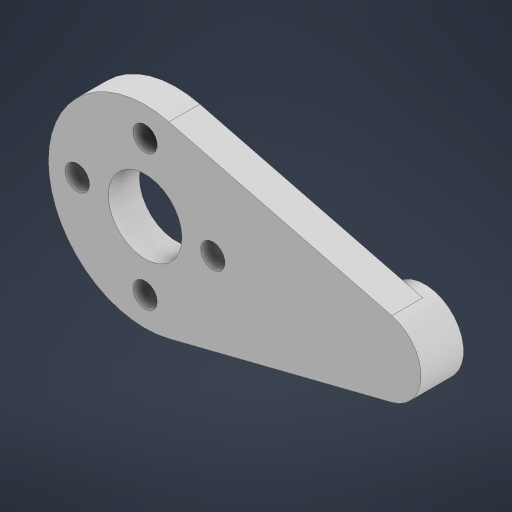
# Autodesk Inventor part: Magnet-arm
Saved by Autodesk Inventor 2024.2 (Build 282272000, 272)
## iProperties
Created: 2024-02-26
Part Number: Magnet-arm
Material: Generisch
Document SubType Name: Modeling
Designer: jacob
Density: 1 g/cm^3
Appearance: Vorgabe
Author: jacob
Autodesk Inventor part; units mm, degrees
ref_plane "YZ Plane" through (0, 0, 0) normal (1, 0, 0) x (0, 1, 0)
ref_plane "XZ Plane" through (0, 0, 0) normal (0, 1, 0) x (-1, 0, 0)
ref_plane "XY Plane" through (0, 0, 0) normal (0, 0, 1) x (1, 0, 0)
sketch "Skizze1" plane through (0, 0, 0) normal (0, 0, 1) x (1, 0, 0)
  arc A0 (2.449, 9.6955) -> (2.449, -9.6955) centre (0, 0) ccw
  arc A1 (25.4796, -3.8782) -> (25.4796, 3.8782) centre (24.5, 0) ccw
  line L0 (25.4796, 3.8782) -> (2.449, 9.6955)
  line L1 (25.4796, -3.8782) -> (2.449, -9.6955)
  circle A2 centre (0, 0) radius 3.8
  dimension "d0" = 20
  dimension "d1" = 8
  dimension "d2" = 24.5
  dimension "d40" = 7.6
  constraints: 4 end point, 4 point on circle, 4 tangent, 3 centre point, 2 coincident, 1 horizontal alignment
  measures "d0" diameter of A0
  measures "d1" diameter of A1
  measures "d2" distance of point (0, 0) A1.centre
  measures "d40" diameter of A2
extrude "Extrusion1" add sketch "Skizze1" along normal blind 3.2
sketch "Skizze2" plane through (0, 0, 0) normal (0, 0, -1) x (-1, 0, 0)
  arc A0 (-25.4796, 3.8782) -> (-25.4796, -3.8782) centre (-24.5, 0) ccw projected
  circle A1 centre (-24.5, 0) radius 4
  point P0 (0, 0)
  point P1 (-25.4796, 3.8782)
  constraints: 1 coincident, 3 other
extrude "Extrusion2" add sketch "Skizze2" along normal blind 1.2
sketch "Skizze3" plane through (24.5, 0, -1.2) normal (0, 0, -1) x (-1, 0, 0)
  circle A0 centre (0, 0) radius 4 projected
  point P0 (24.5, 0)
  constraints: 1 coincident
hole "Bohrung1" at (24.5, 0, -1.2) direction (0, 0, 1) diameter 6.2 depth 2
sketch "Skizze4" plane through (0, 0, 0) normal (0, 0, -1) x (-1, 0, 0)
  point P0 (0, 0)
  point P1 (0, -7)
  dimension "d14" = 7
  constraints: 1 vertical alignment
  measures "d14" distance of point (0, -7) point (0, 0)
hole "Bohrung2" at (0, -7, 0) direction (0, 0, 1) diameter 2.5 end through all
pattern_circular "Runde Anordnung1" count 4 over 360 about axis through (0, 0, 0) along (0, 0, 1) of "Bohrung2"
chamfer "Fasen4" distance 0.2 angle 45 1 edges at (24.5, -3.1, -1.2)
sketch "Skizze5" plane through (24.5, 0, 0.8) normal (0, 0, -1) x (-1, 0, 0)
  circle A0 centre (0, 0) radius 3.1 projected
  point P0 (24.5, 0)
extrude "Extrusion3" cut sketch "Skizze5" against normal blind 0.5
